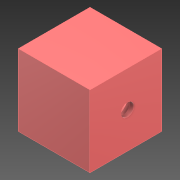
# Autodesk Inventor part: gearbox v2
Saved by Autodesk Inventor 2020 (Build 240168000, 168)
## iProperties
Created: 2020-05-25
Part Number: gearbox v2
Material: Generic
Document SubType Name: Modeling
Designer: stefa
Density: 1 g/cm^3
Appearance: Smooth - Red
Author: stefa
Autodesk Inventor part; units mm, degrees
ref_plane "YZ Plane" through (0, 0, 0) normal (1, 0, 0) x (0, 1, 0)
ref_plane "XZ Plane" through (0, 0, 0) normal (0, 1, 0) x (-1, 0, 0)
ref_plane "XY Plane" through (0, 0, 0) normal (0, 0, 1) x (1, 0, 0)
sketch "Sketch1" plane through (0, 0, 0) normal (0, 0, 1) x (1, 0, 0)
  line L0 (-25, -25) -> (25, -25)
  line L1 (25, -25) -> (25, 25)
  line L2 (25, 25) -> (-25, 25)
  line L3 (-25, 25) -> (-25, -25)
  line L4 (-25, -25) -> (25, 25) construction
  line L5 (25, -25) -> (-25, 25) construction
  line L6 (-15, 15) -> (15, 15)
  line L7 (15, 15) -> (15, -15)
  line L8 (15, -15) -> (-15, -15)
  line L9 (-15, -15) -> (-15, 15)
  circle A0 centre (0, 0) radius 11
  circle A1 centre (0, 0) radius 4.5
  dimension "d0" = 50
  dimension "d1" = 50
  dimension "d2" = 10
  dimension "d3" = 22
  dimension "d4" = 9
  constraints: 20 end point, 4 parallel, 2 centre point, 2 coincident, 2 midpoint, 2 perpendicular, 1 horizontal, 3 other
  measures "d0" distance of L2.end L1.end
  measures "d1" distance of L1.end L0.end
  measures "d2" distance between parallel lines of L2 L6
  measures "d3" diameter of A0
  measures "d4" diameter of A1
extrude "Extrusion1" add sketch "Sketch1" along normal blind 12 contours L3 L2 L1 L0 | L6 L7 L8 L9 | A0 | A1
extrude "Extrusion2" add sketch "Sketch1" against normal blind 38 contours L3 L2 L1 L0
extrude "Extrusion3" cut sketch "Sketch1" along normal blind 7 contours A0
extrude "Extrusion4" cut sketch "Sketch1" along normal blind 10 contours A1
sketch "Sketch3" plane through (15, -15, 0) normal (-1, 0, 0) x (0, 0, 1)
  circle A0 centre (-14.1336, 15) radius 11
  circle A1 centre (-14.1336, 15) radius 4.5
  point P0 (0, 15)
  dimension "d13" = 22
  dimension "d14" = 9
  constraints: 2 centre point, 1 coincident
  measures "d13" diameter of A0
  measures "d14" diameter of A1
extrude "Extrusion5" cut sketch "Sketch3" against normal blind 7
extrude "Extrusion6" cut sketch "Sketch3" against normal through all contours A1
mirror "Mirror1" about plane through (0, 0, 0) normal (1, 0, 0) of "Extrusion5", "Extrusion6"
body "Solid1"
